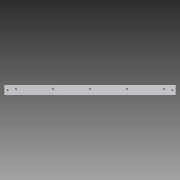
# Autodesk Inventor part: 26in C-Channel Left
Saved by Autodesk Inventor 2013 (Build 170138000, 138)
## iProperties
Created: 2013-01-08
Part Number: 26in C-Channel Left
Material: Aluminum 6061
Document SubType Name: Modeling
Designer: Naphat
Density: 2.71 g/cm^3
Mass: 343.469 g
Surface Area: 887.22 cm^2
Volume: 126.741 cm^3
Author: Naphat
Autodesk Inventor part; units mm, degrees
ref_plane "YZ Plane" through (0, 0, 0) normal (1, 0, 0) x (0, 1, 0)
ref_plane "XZ Plane" through (0, 0, 0) normal (0, 1, 0) x (-1, 0, 0)
ref_plane "XY Plane" through (0, 0, 0) normal (0, 0, 1) x (1, 0, 0)
sketch "Sketch1" plane through (0, 0, 0) normal (0, 0, 1) x (1, 0, 0)
  line L0 (-16, 12.5) -> (-13, 12.5)
  line L1 (-13, 12.5) -> (-13, -9.5)
  line L2 (-13, -9.5) -> (13, -9.5)
  line L3 (13, -9.5) -> (13, 12.5)
  line L4 (13, 12.5) -> (16, 12.5)
  line L5 (16, 12.5) -> (16, -12.5)
  line L6 (16, -12.5) -> (-16, -12.5)
  line L7 (-16, -12.5) -> (-16, 12.5)
  point P0 (0, 0)
  dimension "d0" = 3
  dimension "d2" = 3
  dimension "d3" = 25
  dimension "d4" = 32
  dimension "d5" = 16
  dimension "d7" = 12.5
  dimension "d8" = 3
  dimension "d95" = 25
  constraints: 16 end point, 5 parallel, 1 collinear, 1 horizontal, 1 perpendicular
  measures "d0" distance of L0.start L0.end
  measures "d2" distance of L3.end L4.end
  measures "d3" distance of L6.end L0.start
  measures "d4" distance of L5.end L6.end
  measures "d5" distance from line of point (0, 0) L7
  measures "d7" distance from line of L6 point (0, 0)
  measures "d8" distance between parallel lines of L6 L2
  measures "d95" distance between parallel lines of L6 L4
extrude "Extrusion1" add sketch "Sketch1" against normal blind 558.8
sketch "Sketch7" plane through (-16, -12.5, 0) normal (0, -1, 0) x (1, 0, 0)
  line L0 (32, 0) -> (0, 0) projected
  line L1 (32, -558.8) -> (0, -558.8) projected
  line L2 (32, 0) -> (32, -558.8) projected
  circle A0 centre (16, -11) radius 3.175
  circle A1 centre (16, -547.8) radius 3.175
  point P0 (16, 0)
  dimension "d103" = 6.35
  dimension "d104" = 11
  dimension "d105" = 16
  dimension "d106" = 6.35
  dimension "d108" = 16
  dimension "d109" = 11
  constraints: 2 centre point
  measures "d103" diameter of A0
  measures "d104" distance from line of A0.centre L0
  measures "d105" distance from line of L2 A0.centre
  measures "d106" diameter of A1
  measures "d108" distance from line of A1.centre L2
  measures "d109" distance from line of A1.centre L1
hole "Hole3" at (0, -12.5, -547.8) at (0, -12.5, -11) direction (0, 1, 0) diameter 6.35 end through all
sketch "Sketch8" plane through (-16, -12.5, 0) normal (0, -1, 0) x (1, 0, 0)
  line L0 (12.7, -35.2242) -> (34.3, -35.2242) construction
  arc A0 (12.7, -276.4246) -> (12.7, -282.7746) centre (12.7, -279.5996) ccw construction
  line L1 (12.7, -276.4246) -> (34.3, -276.4246) construction
  arc A1 (34.3, -282.7746) -> (34.3, -276.4246) centre (34.3, -279.5996) ccw construction
  line L2 (34.3, -282.7746) -> (12.7, -282.7746) construction
  arc A2 (12.7, -155.8244) -> (12.7, -162.1744) centre (12.7, -158.9994) ccw construction
  line L3 (12.7, -155.8244) -> (34.3, -155.8244) construction
  arc A3 (34.3, -162.1744) -> (34.3, -155.8244) centre (34.3, -158.9994) ccw construction
  line L4 (34.3, -162.1744) -> (12.7, -162.1744) construction
  arc A4 (34.3, -523.975) -> (34.3, -517.625) centre (34.3, -520.8) ccw construction
  line L5 (34.3, -523.975) -> (12.7, -523.975) construction
  arc A5 (12.7, -517.625) -> (12.7, -523.975) centre (12.7, -520.8) ccw construction
  line L6 (12.7, -517.625) -> (34.3, -517.625) construction
  arc A6 (12.7, -397.0248) -> (12.7, -403.3748) centre (12.7, -400.1998) ccw construction
  line L7 (12.7, -397.0248) -> (34.3, -397.0248) construction
  arc A7 (34.3, -403.3748) -> (34.3, -397.0248) centre (34.3, -400.1998) ccw construction
  line L8 (34.3, -403.3748) -> (12.7, -403.3748) construction
  arc A8 (34.3, -41.5742) -> (34.3, -35.2242) centre (34.3, -38.3992) ccw construction
  line L9 (34.3, -41.5742) -> (12.7, -41.5742) construction
  arc A9 (12.7, -35.2242) -> (12.7, -41.5742) centre (12.7, -38.3992) ccw construction
  line L10 (12.7, -35.2242) -> (34.3, -35.2242) construction
  line L11 (47, -22.3992) -> (0, -22.3992) construction
  line L12 (0, -22.3992) -> (0, -536.8) construction
  line L13 (47, -536.8) -> (0, -536.8) construction
  line L14 (47, -22.3992) -> (47, -536.8) construction
  circle A10 centre (12.7, -38.3992) radius 3.175
  circle A11 centre (12.7, -158.9994) radius 3.175
  circle A12 centre (12.7, -279.5996) radius 3.175
  circle A13 centre (12.7, -400.1998) radius 3.175
  circle A14 centre (12.7, -520.8) radius 3.175
  point P0 (16, 0)
  constraints: 5 coincident, 5 vertical alignment, 10 other
hole "Hole4" at (-3.3, -12.5, -38.3992) at (-3.3, -12.5, -158.9994) at (-3.3, -12.5, -279.5996) at (-3.3, -12.5, -400.1998) at (-3.3, -12.5, -520.8) direction (0, 1, 0) diameter 6.35 depth 3 tip angle 118
equation "\"d2\" = d0"
equation "\"d5\" = 0.5 * d4"
equation "\"d7\" = 0.5 * d3"
equation "\"d8\" = d0"
equation "\"d95\" = d3"
body "Solid1"
